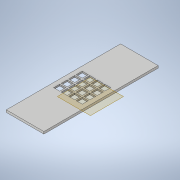
# Autodesk Inventor part: scope coverslip holder lowpro offset
Saved by Autodesk Inventor 2022 (Build 260153000, 153)
## iProperties
Created: 2019-09-11
Part Number: scope coverslip holder lowpro offset
Material: Generic
Document SubType Name: Modeling
Designer: Eamon
Density: 1 g/cm^3
Appearance: Default
Author: Eamon
Autodesk Inventor part; units mm, degrees
ref_plane "YZ Plane" through (0, 0, 0) normal (1, 0, 0) x (0, 1, 0)
ref_plane "XZ Plane" through (0, 0, 0) normal (0, 1, 0) x (-1, 0, 0)
ref_plane "XY Plane" through (0, 0, 0) normal (0, 0, 1) x (1, 0, 0)
sketch "Sketch1" plane through (0, 0, 0) normal (0, 1, 0) x (-1, 0, 0)
  line L0 (0, 0) -> (25, 0)
  line L1 (25, 0) -> (25, -76)
  line L2 (25, -76) -> (0, -76)
  line L3 (0, -76) -> (0, 0)
  dimension "d0" = 76
  dimension "d1" = 25
  constraints: 8 end point, 2 parallel, 1 horizontal, 1 perpendicular
  measures "d0" distance of L2.end L0.start
  measures "d1" distance of L0.start L0.end
extrude "Extrusion1" add sketch "Sketch1" along normal blind 1.5
ref_plane "Work Plane2" through (0, 5.5, 0) normal (0, 1, 0) x (1, 0, 0)
sketch "Sketch3" plane through (0, 5.5, 0) normal (0, 1, 0) x (1, 0, 0)
  line L0 (0, 0) -> (-25, 0) construction
  line L1 (-12.5, 0) -> (-12.5, 76) construction
  line L2 (-25, 76) -> (0, 76) construction
  line L3 (-25, 71) -> (-25, 5) construction
  line L4 (-25, 38) -> (-0.4405, 38) construction
  line L5 (-20, 28.5) -> (-5, 28.5) construction
  line L6 (-3, 30.5) -> (-3, 45.5) construction
  line L7 (-5, 47.5) -> (-20, 47.5) construction
  line L8 (-22, 45.5) -> (-22, 30.5) construction
  line L9 (-22, 28.5) -> (-3, 47.5) construction
  line L10 (-3, 28.5) -> (-22, 47.5) construction
  arc A0 (-20, 47.5) -> (-22, 45.5) centre (-20, 45.5) ccw construction
  arc A1 (-3, 45.5) -> (-5, 47.5) centre (-5, 45.5) ccw construction
  arc A2 (-5, 28.5) -> (-3, 30.5) centre (-5, 30.5) ccw construction
  arc A3 (-22, 30.5) -> (-20, 28.5) centre (-20, 30.5) ccw construction
  line L11 (-22, 47.5) -> (-18, 47.5)
  line L12 (-18, 47.5) -> (-18, 43.5)
  line L13 (-18, 43.5) -> (-22, 43.5)
  line L14 (-22, 43.5) -> (-22, 47.5)
  line L15 (0, 47.5) -> (-15, 47.5) construction
  line L16 (-13, 43.5) -> (-17, 43.5)
  line L17 (-13, 47.5) -> (-13, 43.5)
  line L18 (-17, 47.5) -> (-13, 47.5)
  line L19 (-17, 43.5) -> (-17, 47.5)
  line L20 (5, 47.5) -> (-10, 47.5) construction
  line L21 (-8, 43.5) -> (-12, 43.5)
  line L22 (-8, 47.5) -> (-8, 43.5)
  line L23 (-12, 47.5) -> (-8, 47.5)
  line L24 (-12, 43.5) -> (-12, 47.5)
  line L25 (10, 47.5) -> (-5, 47.5) construction
  line L26 (-3, 43.5) -> (-7, 43.5)
  line L27 (-3, 47.5) -> (-3, 43.5)
  line L28 (-7, 47.5) -> (-3, 47.5)
  line L29 (-7, 43.5) -> (-7, 47.5)
  line L30 (-5, 42.5) -> (-20, 42.5) construction
  line L31 (-18, 38.5) -> (-22, 38.5)
  line L32 (-18, 42.5) -> (-18, 38.5)
  line L33 (-22, 42.5) -> (-18, 42.5)
  line L34 (-22, 38.5) -> (-22, 42.5)
  line L35 (0, 42.5) -> (-15, 42.5) construction
  line L36 (-13, 38.5) -> (-17, 38.5)
  line L37 (-13, 42.5) -> (-13, 38.5)
  line L38 (-17, 42.5) -> (-13, 42.5)
  line L39 (-17, 38.5) -> (-17, 42.5)
  line L40 (5, 42.5) -> (-10, 42.5) construction
  line L41 (-8, 38.5) -> (-12, 38.5)
  line L42 (-8, 42.5) -> (-8, 38.5)
  line L43 (-12, 42.5) -> (-8, 42.5)
  line L44 (-12, 38.5) -> (-12, 42.5)
  line L45 (10, 42.5) -> (-5, 42.5) construction
  line L46 (-3, 38.5) -> (-7, 38.5)
  line L47 (-3, 42.5) -> (-3, 38.5)
  line L48 (-7, 42.5) -> (-3, 42.5)
  line L49 (-7, 38.5) -> (-7, 42.5)
  line L50 (-5, 37.5) -> (-20, 37.5) construction
  line L51 (-18, 33.5) -> (-22, 33.5)
  line L52 (-18, 37.5) -> (-18, 33.5)
  line L53 (-22, 37.5) -> (-18, 37.5)
  line L54 (-22, 33.5) -> (-22, 37.5)
  line L55 (0, 37.5) -> (-15, 37.5) construction
  line L56 (-13, 33.5) -> (-17, 33.5)
  line L57 (-13, 37.5) -> (-13, 33.5)
  line L58 (-17, 37.5) -> (-13, 37.5)
  line L59 (-17, 33.5) -> (-17, 37.5)
  line L60 (5, 37.5) -> (-10, 37.5) construction
  line L61 (-8, 33.5) -> (-12, 33.5)
  line L62 (-8, 37.5) -> (-8, 33.5)
  line L63 (-12, 37.5) -> (-8, 37.5)
  line L64 (-12, 33.5) -> (-12, 37.5)
  line L65 (10, 37.5) -> (-5, 37.5) construction
  line L66 (-3, 33.5) -> (-7, 33.5)
  line L67 (-3, 37.5) -> (-3, 33.5)
  line L68 (-7, 37.5) -> (-3, 37.5)
  line L69 (-7, 33.5) -> (-7, 37.5)
  line L70 (-5, 32.5) -> (-20, 32.5) construction
  line L71 (-18, 28.5) -> (-22, 28.5)
  line L72 (-18, 32.5) -> (-18, 28.5)
  line L73 (-22, 32.5) -> (-18, 32.5)
  line L74 (-22, 28.5) -> (-22, 32.5)
  line L75 (0, 32.5) -> (-15, 32.5) construction
  line L76 (-13, 28.5) -> (-17, 28.5)
  line L77 (-13, 32.5) -> (-13, 28.5)
  line L78 (-17, 32.5) -> (-13, 32.5)
  line L79 (-17, 28.5) -> (-17, 32.5)
  line L80 (5, 32.5) -> (-10, 32.5) construction
  line L81 (-8, 28.5) -> (-12, 28.5)
  line L82 (-8, 32.5) -> (-8, 28.5)
  line L83 (-12, 32.5) -> (-8, 32.5)
  line L84 (-12, 28.5) -> (-12, 32.5)
  line L85 (10, 32.5) -> (-5, 32.5) construction
  line L86 (-3, 28.5) -> (-7, 28.5)
  line L87 (-3, 32.5) -> (-3, 28.5)
  line L88 (-7, 32.5) -> (-3, 32.5)
  line L89 (-7, 28.5) -> (-7, 32.5)
  point P0 (-12.5, 38)
  point P1 (2, 47.5)
  point P2 (7, 47.5)
  point P3 (12, 47.5)
  point P4 (-3, 42.5)
  point P5 (2, 42.5)
  point P6 (7, 42.5)
  point P7 (12, 42.5)
  point P8 (-3, 37.5)
  point P9 (2, 37.5)
  point P10 (7, 37.5)
  point P11 (12, 37.5)
  point P12 (-3, 32.5)
  point P13 (2, 32.5)
  point P14 (7, 32.5)
  point P15 (12, 32.5)
  dimension "d8" = 19
  dimension "d9" = 2
  dimension "d10" = 2
  dimension "d11" = 2
  dimension "d12" = 2
  dimension "d20" = 4
  dimension "d23" = 5
  dimension "d26" = 5
  constraints: 174 end point, 40 point on line, 8 point on circle, 8 tangent, 6 midpoint, 4 centre point, 4 parallel, 3 horizontal, 3 perpendicular, 2 vertical, 1 collinear, 179 other
  measures "d8" distance of L9.end L10.end
  measures "d9" radius of A0
  measures "d10" radius of A1
  measures "d11" radius of A2
  measures "d12" radius of A3
  measures "d20" distance of L11.end L12.end
  measures "d23" distance of L7.start L15.start
  measures "d26" distance of L7.start L30.start
extrude "Extrusion3" cut sketch "Sketch3" against normal blind 6
sketch "Sketch4" plane through (0, 0, 0) normal (0, -1, 0) x (1, 0, 0)
  line L0 (0, -76) -> (0, 0) construction
  line L1 (0, -38) -> (-25, -38) construction
  line L2 (-25, -71) -> (-25, -5) construction
  line L3 (0, 0) -> (-25, 0) construction
  line L4 (-12.5, 0) -> (-12.5, -76) construction
  line L5 (-25, -76) -> (0, -76) construction
  line L6 (-19.875, -49.375) -> (-5.125, -49.375)
  line L7 (-1.125, -49.375) -> (-1.125, -26.625)
  line L8 (-5.125, -26.625) -> (-19.875, -26.625)
  line L9 (-23.875, -26.625) -> (-23.875, -49.375)
  line L10 (-23.875, -49.375) -> (-1.125, -26.625) construction
  line L11 (-1.125, -49.375) -> (-23.875, -26.625) construction
  arc A0 (-1.125, -26.625) -> (-5.125, -26.625) centre (-3.125, -26.625) ccw
  arc A1 (-19.875, -26.625) -> (-23.875, -26.625) centre (-21.875, -26.625) ccw
  arc A2 (-23.875, -49.375) -> (-19.875, -49.375) centre (-21.875, -49.375) ccw
  arc A3 (-5.125, -49.375) -> (-1.125, -49.375) centre (-3.125, -49.375) ccw
  point P0 (-12.5, -38)
  dimension "d15" = 22.75
  dimension "d16" = 4
  dimension "d17" = 22.75
  constraints: 16 end point, 8 point on circle, 7 midpoint, 4 centre point, 4 point on line, 4 vertical alignment, 3 equal radius, 3 horizontal alignment, 2 parallel, 1 horizontal, 1 perpendicular, 1 tangent
  measures "d15" distance of L7.end L9.start
  measures "d16" diameter of A0
  measures "d17" distance of L7.start L7.end
extrude "Extrusion4" cut sketch "Sketch4" against normal blind 0.5
body "Solid1"
